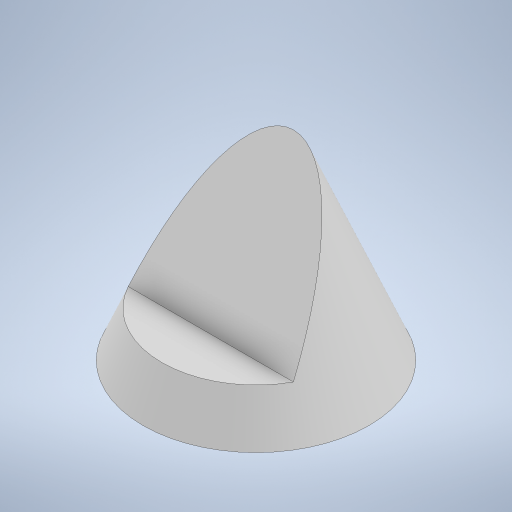
# Autodesk Inventor part: 20
Saved by Autodesk Inventor 2024 (Build 280153000, 153)
## iProperties
Created: 2023-11-17
Part Number: 20
Material: Типовые
Document SubType Name: Modeling
Designer: User
Density: 1 g/cm^3
Appearance: По умолчанию
Author: User
Autodesk Inventor part; units mm, degrees
ref_plane "YZ Plane" through (0, 0, 0) normal (1, 0, 0) x (0, 1, 0)
ref_plane "XZ Plane" through (0, 0, 0) normal (0, 1, 0) x (-1, 0, 0)
ref_plane "XY Plane" through (0, 0, 0) normal (0, 0, 1) x (1, 0, 0)
sketch "Эскиз1" plane through (0, 0, 0) normal (1, 0, 0) x (0, 1, 0)
  line L0 (0, 0) -> (120, 0)
  line L1 (120, 0) -> (0, -50)
  line L2 (0, -50) -> (0, 0)
  dimension "d0" = 50
  dimension "d1" = 120
  constraints: 6 end point, 1 horizontal, 1 perpendicular
  measures "d0" distance of L1.end L0.start
  measures "d1" distance of L0.start L0.end
revolve "Вращение1" add sketch "Эскиз1" angle 360 about axis through (0, 0, 0) along (0, 1, 0)
sketch "Эскиз2" plane through (0, 0, 0) normal (1, 0, 0) x (0, 1, 0)
  line L0 (0, -50) -> (120, 0) projected
  line L1 (0, 50) -> (120, 0) projected
  line L2 (20, 41.6667) -> (20, 20)
  line L3 (0, -50) -> (0, 50) projected
  line L4 (80, -16.6667) -> (20, 20)
  point P0 (0, 0)
  constraints: 4 end point, 2 point on line
extrude "Выдавливание1" cut sketch "Эскиз2" along normal mid plane 200 contours L4 L2 L1 L0
